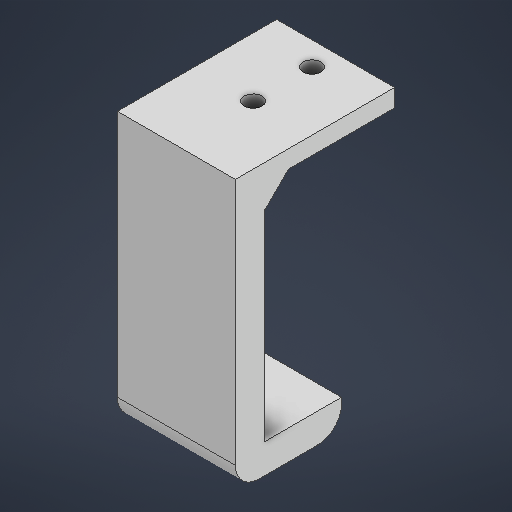
# Autodesk Inventor part: Front_Skit_Plate
Saved by Autodesk Inventor 2026.1 (Build 301233020, 233B)
## iProperties
Created: 2025-10-16
Part Number: Front_Skit_Plate
Material: Generic
Document SubType Name: Modeling
Designer: Garfieldcmix
Density: 1 g/cm^3
Appearance: Default
Author: Garfieldcmix
Autodesk Inventor part; units mm, degrees
ref_plane "YZ Plane" through (0, 0, 0) normal (1, 0, 0) x (0, 1, 0)
ref_plane "XZ Plane" through (0, 0, 0) normal (0, 1, 0) x (-1, 0, 0)
ref_plane "XY Plane" through (0, 0, 0) normal (0, 0, 1) x (1, 0, 0)
sketch "Sketch1" plane through (0, 0, 0) normal (1, 0, 0) x (0, 1, 0)
  line L0 (0, 0) -> (-46, 0)
  line L1 (-46, 0) -> (-46, -18)
  line L2 (-46, -18) -> (-41, -18)
  line L3 (-41, -18) -> (-41, -5)
  line L4 (-41, -5) -> (-3, -5)
  line L5 (-3, -5) -> (-3, -27)
  line L6 (-3, -27) -> (0, -27)
  line L7 (0, -27) -> (0, 0)
  dimension "d0" = 3
  dimension "d1" = 46
  dimension "d2" = 5
  dimension "d3" = 27
  dimension "d4" = 18
  dimension "d5" = 5
  constraints: 16 end point, 7 perpendicular, 1 horizontal
  measures "d0" distance of L5.end L6.end
  measures "d1" distance of L0.start L0.end
  measures "d2" distance between parallel lines of L4 L0
  measures "d3" distance of L6.end L0.start
  measures "d4" distance of L0.end L1.end
  measures "d5" distance of L1.end L2.end
extrude "Extrusion1" add sketch "Sketch1" along normal blind 20
fillet "Fillet1" radius 4 2 edges at (10, -46, 0) (10, -46, -18)
chamfer "Chamfer1" distance 4 angle 45 1 edges at (10, -3, -5)
sketch "Sketch2" plane through (0, 0, 0) normal (0, 1, 0) x (1, 0, 0)
  circle A0 centre (10, 13) radius 1.5
  circle A1 centre (10, 23) radius 1.5
  line L0 (0, 0) -> (20, 0) construction
  line L1 (10, 0) -> (10, 27) construction
  line L2 (0, 27) -> (20, 27) construction
  dimension "d12" = 3
  dimension "d13" = 13
  dimension "d14" = 10
  constraints: 2 centre point, 2 end point, 2 midpoint, 2 point on line, 1 equal radius
  measures "d12" diameter of A0
  measures "d13" distance from line of L0 A0.centre
  measures "d14" distance of A1.centre A0.centre
extrude "Extrusion2" cut sketch "Sketch2" against normal up to surface (3 mm away)
body "Solid1"
